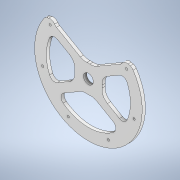
# Autodesk Inventor part: TH22_POM_X
Saved by Autodesk Inventor 2022 (Build 260153000, 153)
## iProperties
Created: 2021-12-06
Part Number: TH22_POM_X
Material: ABS プラスチック
Document SubType Name: Modeling
Designer: 中島 青蔵
Density: 1.06 g/cm^3
Appearance: 滑らか - 白
Author: 中島 青蔵
Autodesk Inventor part; units mm, degrees
ref_plane "YZ Plane" through (0, 0, 0) normal (1, 0, 0) x (0, 1, 0)
ref_plane "XZ Plane" through (0, 0, 0) normal (0, 1, 0) x (-1, 0, 0)
ref_plane "XY Plane" through (0, 0, 0) normal (0, 0, 1) x (1, 0, 0)
sketch "スケッチ1" plane through (0, 0, 0) normal (0, 0, 1) x (1, 0, 0)
  circle A0 centre (69, 50) radius 2
  circle A1 centre (0, 0) radius 9
  circle A2 centre (0, 0) radius 25
  circle A3 centre (69, 50) radius 7.5
  line L0 (65.25, 56.4952) -> (8.2643, 23.5945)
  line L1 (0, 25) -> (0, -25)
  line L2 (-25, 0) -> (25, 0)
  line L3 (20.9707, 13.61) -> (72.75, 43.5048)
  circle A4 centre (69, -50) radius 2
  circle A5 centre (69, -50) radius 7.5
  line L4 (65.25, -56.4952) -> (8.2643, -23.5945)
  line L5 (20.9707, -13.61) -> (72.75, -43.5048)
  circle A6 centre (-69, 50) radius 2
  circle A7 centre (-69, 50) radius 7.5
  line L6 (-65.25, 56.4952) -> (-8.2643, 23.5945)
  line L7 (-20.9707, 13.61) -> (-72.75, 43.5048)
  line L8 (-65.25, -56.4952) -> (-8.2643, -23.5945)
  circle A8 centre (-69, -50) radius 7.5
  circle A9 centre (-69, -50) radius 2
  line L9 (-20.9707, -13.61) -> (-72.75, -43.5048)
  circle A10 centre (0, 0) radius 77
  circle A11 centre (0, 0) radius 86.5
  circle A12 centre (0, 0) radius 98.5
  line L10 (0, 0) -> (79.6882, 57.8968)
  line L11 (0, 0) -> (95.4054, -24.496)
  line L12 (0, 0) -> (41.9393, -89.1255)
  line L13 (0, 0) -> (-79.6882, 57.8968)
  line L14 (0, 0) -> (-95.4054, -24.496)
  line L15 (0, 0) -> (-41.9393, -89.1255)
  circle A13 centre (69.98, 50.8434) radius 2
  circle A14 centre (83.7824, -21.5117) radius 2
  circle A15 centre (36.8299, -78.2675) radius 2
  circle A16 centre (69.98, 50.8434) radius 9.5
  circle A17 centre (-69.98, 50.8434) radius 2
  circle A18 centre (-83.7824, -21.5117) radius 2
  circle A19 centre (-36.8299, -78.2675) radius 2
  circle A20 centre (-69.98, 50.8434) radius 9.5
  line L16 (-79.6882, 57.8968) -> (-72.6529, 59.9596)
  line L17 (79.6882, 57.8968) -> (72.6529, 59.9596)
  point P0 (-8.2643, 23.5945)
  point P1 (-8.2643, -23.5945)
  point P2 (8.2643, -23.5945)
  point P3 (66.0238, -39.6214)
  point P4 (57.0218, -51.7447)
  point P5 (-57.0218, -51.7447)
  point P6 (-66.0238, -39.6214)
  point P7 (-66.0238, 39.6214)
  point P8 (-57.0218, 51.7447)
  point P9 (-62.2943, 45.2595)
  point P10 (-77.6656, 56.4274)
  point P11 (77.6656, 56.4274)
  point P12 (62.2943, 45.2595)
  point P13 (57.0218, 51.7447)
  point P14 (66.0238, 39.6214)
  point P15 (-61.0434, 54.0665)
  point P16 (61.0434, 54.0665)
  point P17 (69.0803, 41.3861)
  point P18 (-69.0803, 41.3861)
  point P19 (-12.1615, -25.8445)
  point P20 (-10.6445, -22.6207)
  point P21 (10.6445, -22.6207)
  point P22 (12.1615, -25.8445)
  dimension "d19" = 19
  dimension "d0" = 4
  dimension "d1" = 50
  dimension "d2" = 69
  dimension "d3" = 18
  dimension "d4" = 50
  dimension "d5" = 15
  dimension "d6" = 30
  dimension "d10" = 154
  dimension "d11" = 173
  dimension "d12" = 197
  dimension "d13" = 54
  dimension "d14" = 50.4
  dimension "d15" = 50.4
  dimension "d16" = 4
  dimension "d17" = 4
  dimension "d18" = 4
  constraints: 36 end point, 25 symmetric about line, 20 point on circle, 19 centre point, 11 coincident, 3 point on line, 2 tangent, 2 vertical, 1 horizontal, 1 parallel, 17 other
  measures "d0" diameter of A0
  measures "d1" vertical distance of point (0, 0) A0.centre
  measures "d2" horizontal distance of point (0, 0) A0.centre
  measures "d3" diameter of A1
  measures "d4" diameter of A2
  measures "d5" diameter of A3
  measures "d6" angle of L2 L0
  measures "d10" diameter of A10
  measures "d11" diameter of A11
  measures "d12" diameter of A12
  measures "d13" angle of L1 L10
  measures "d14" angle of L10 L11
  measures "d15" angle of L12 L11
  measures "d16" diameter of A13
  measures "d17" diameter of A14
  measures "d18" diameter of A15
extrude "押し出し1" add sketch "スケッチ1" along normal blind 5.8 contours A13 A11 A3 L10 | L10 A3 A11 A13 | A13 A11 A3 L10 A0 | A0 L10 A13 | A13 L10 A0 | A0 L10 A3 A11 A13 | L10 A16 A11 A3 | A3 A11 A16 L10 | A11 A16 L3 A3 | A3 L0 A16 A11 | A16 L17 L10 | L10 A12 L11 A14 A11 A16 | L10 A16 L0 A3 | A3 L3 A16 L10 | A11 A14 L11 A10 L3 A16 | A16 L3 A10 | L10 A2 L0 A10 | A10 L3 A2 L10 | A10 L0 A16 | A20 L6 A7 A11 | A11 A7 L13 A20 | L13 A20 A11 A18 L14 A12 | L16 A20 L13 | L10 A1 L1 A2 | A2 L2 A1 L10 | A11 A17 L13 A7 | A7 L13 A6 A17 A11 | A20 L13 A7 L6 | L6 A10 A20 | A12 L12 A15 A11 A5 A14 L11 | L14 A18 A11 A8 A19 L15 A12 | L13 A7 A11 A20 | L6 A2 L13 A10 | A14 A11 A5 L5 A10 L11 | L13 A17 A11 A7 | A12 L15 A19 A11 A15 L12 | A20 L7 A10 L14 A18 A11 | A11 A7 L7 A20 | A2 L11 A1 L2 | L1 A1 L13 A2 | L13 A2 L7 A10 | A20 L7 A7 L13 | A10 L7 A20 | A11 A17 A6 L13 A7 | A6 L13 A17 | A18 L14 A10 L9 A8 A11 | A2 L12 A1 L11 | A10 L4 L12 A2 L5 | L5 A5 L4 A10 | L13 A1 L2 A2 | L1 A2 L15 A1 | A1 L12 A2 L1 | A1 L14 A2 L2 | A1 L15 A2 L14 | A11 A4 A5 | A5 A11 A4 | A11 A19 L15 A10 L12 A15 | A11 A8 L8 A10 L15 A19 | A11 A9 A8 | A8 A11 A9 | L4 A5 A11 A15 L12 A10 | A6 A17 L13 | L12 L4 A2 | L15 L8 A10 L9 A2 | A2 L8 L15 | A11 A4 | A4 A11 | L9 A10 L8 A8 | A11 A9 | A9 A11
fillet "フィレット1" radius 20 8 edges at (-8.2643, 23.5945, 2.9) (8.2643, 23.5945, 2.9) (-8.2643, -23.5945, 2.9) (8.2643, -23.5945, 2.9) (-20.9707, -13.61, 2.9) (-20.9707, 13.61, 2.9) (20.9707, 13.61, 2.9) (20.9707, -13.61, 2.9)
fillet "フィレット2" radius 10 10 edges at (-61.0434, 54.0665, 2.9) (61.0434, 54.0665, 2.9) (66.0238, 39.6214, 2.9) (66.0238, -39.6214, 2.9) (57.0218, -51.7447, 2.9) (-57.0218, -51.7447, 2.9) (-66.0238, -39.6214, 2.9) (-66.0238, 39.6214, 2.9) (79.6882, 57.8968, 2.9) (-79.6882, 57.8968, 2.9)
equation "\"d15\" = d14"
